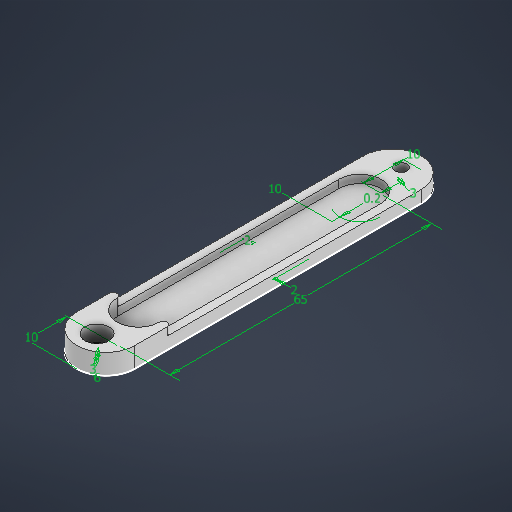
# Autodesk Inventor part: magnet_holder
Saved by Autodesk Inventor 2026.2 (Build 302298000, 298)
## iProperties
Created: 2026-03-09
Part Number: magnet_holder
Material: Generic
Document SubType Name: Modeling
Designer: Tathagata Sikdar
Density: 1 g/cm^3
Appearance: Default
Author: Tathagata Sikdar
Autodesk Inventor part; units mm, degrees
ref_plane "YZ Plane" through (0, 0, 0) normal (1, 0, 0) x (0, 1, 0)
ref_plane "XZ Plane" through (0, 0, 0) normal (0, 1, 0) x (-1, 0, 0)
ref_plane "XY Plane" through (0, 0, 0) normal (0, 0, 1) x (1, 0, 0)
sketch "Sketch1" plane through (0, 0, 0) normal (0, 1, 0) x (-1, 0, 0)
  line L0 (0, 0) -> (0, -65) construction
  line L1 (-5, -5) -> (-5, -60) construction
  line L2 (5, -60) -> (5, -5) construction
  arc A0 (5, -5) -> (-5, -5) centre (0, -5) ccw construction
  arc A1 (-5, -60) -> (5, -60) centre (0, -60) ccw construction
  line L3 (5.2, -60) -> (5.2, -5)
  arc A2 (5.2, -5) -> (-5.2, -5) centre (0, -5) ccw
  line L4 (-5.2, -5) -> (-5.2, -60)
  arc A3 (-5.2, -60) -> (5.2, -60) centre (0, -60) ccw
  arc A4 (7.2, 3) -> (-7.2, 3) centre (0, 3) ccw
  line L5 (-7.2, 3) -> (-7.2, -68)
  arc A5 (-7.2, -68) -> (7.2, -68) centre (0, -68) ccw
  line L6 (7.2, -68) -> (7.2, 3)
  circle A6 centre (0, -70.2) radius 1.5
  line L7 (0, -75.2) -> (0, -65.2) construction
  circle A7 centre (0, 5.2) radius 1.5
  line L8 (0, 0.2) -> (0, 10.2) construction
  circle A8 centre (0, 5.2) radius 3
  arc A9 (-7.2, -5) -> (-5.2, -5) centre (-6.2, -5) ccw
  arc A10 (5.2, -5) -> (7.2, -5) centre (6.2, -5) ccw
  point P0 (0, -32.5)
  point P1 (7.2, -32.5)
  point P2 (0, -70.2)
  dimension "d0" = 65
  dimension "d1" = 10
  dimension "d2" = 0.2
  dimension "d8" = 2
  dimension "d9" = 2
  dimension "d10" = 10
  dimension "d11" = 10
  dimension "d12" = 3
  dimension "d13" = 3
  dimension "d14" = 6
  constraints: 22 point on circle, 20 end point, 12 tangent, 11 centre point, 4 midpoint, 4 point on line, 4 vertical, 3 coincident, 2 parallel, 3 other
  measures "d0" distance of L0.start L0.end
  measures "d1" diameter of A1
  measures "d2" radial gap between concentric circles of A1 A3
  measures "d8" distance between parallel lines of L5 L4
  measures "d9" distance from line of point (7.2, -32.5) L3
  measures "d10" distance of L7.start L7.end
  measures "d11" distance of L8.end L8.start
  measures "d12" diameter of A6
  measures "d13" diameter of A7
  measures "d14" diameter of A8
extrude "Extrusion3" add sketch "Sketch1" along normal blind 1 contours A3 L4 A2 L3 | L3 A10 L6 A5 L5 A9 L4 A3 | A2 A9 L5 A4 L6 A10 | A8
extrude "Extrusion4" add sketch "Sketch1" along normal blind 2 from surface at 1 contours L3 A10 L6 A5 L5 A9 L4 A3 | A2 A9 L5 A4 L6 A10
extrude "Extrusion5" add sketch "Sketch1" along normal blind 2 from surface at 3 contours A2 A9 L5 A4 L6 A10
body "Solid2"
